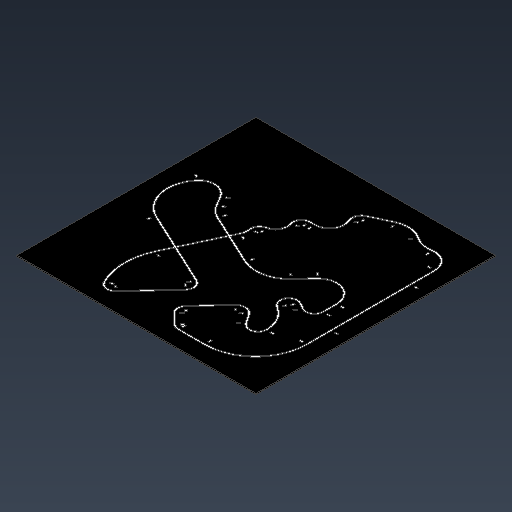
# Autodesk Inventor part: Pista_V2
Saved by Autodesk Inventor 2026.1 (Build 301233020, 233B)
## iProperties
Created: 2026-03-26
Part Number: Pista_V2
Material: Genérico
Document SubType Name: Modeling
Designer: celio
Density: 1 g/cm^3
Appearance: Padrão
Author: celio
Autodesk Inventor part; units mm, degrees
(part 1 of 2)
ref_plane "YZ Plane" through (0, 0, 0) normal (1, 0, 0) x (0, 1, 0)
ref_plane "XZ Plane" through (0, 0, 0) normal (0, 1, 0) x (-1, 0, 0)
ref_plane "XY Plane" through (0, 0, 0) normal (0, 0, 1) x (1, 0, 0)
sketch "Esboço3" plane through (0, 0, 0) normal (0, 1, 0) x (-1, 0, 0)
  line L0 (0, 0) -> (3000, 0)
  line L1 (3000, 0) -> (3000, 3000)
  line L2 (3000, 3000) -> (0, 3000)
  line L3 (0, 3000) -> (0, 0)
  line L4 (2800, 200) -> (200, 200)
  line L5 (200, 200) -> (200, 2800)
  line L6 (200, 2800) -> (2800, 2800)
  line L7 (2800, 2800) -> (2800, 200)
  dimension "d59" = 3000
  dimension "d60" = 3000
  dimension "d62" = 200
  constraints: 16 end point, 4 parallel, 2 perpendicular, 1 horizontal, 3 other
  measures "d59" distance of L2.end L1.end
  measures "d60" distance of L1.end L0.end
  measures "d62" distance between parallel lines of L0 L4
sketch "Esboço2" plane through (0, 0, 0) normal (0, 1, 0) x (-1, 0, 0)
  line L0 (203.1812, 1286.807) -> (200.7366, 822.1752)
  line L1 (200.7366, 822.1752) -> (213.5115, 423.3861)
  arc A0 (213.5115, 423.3861) -> (413.6397, 320.4728) centre (342.1557, 427.5072) ccw
  arc A1 (570.2436, 314.2066) -> (413.6397, 320.4728) centre (487.6339, 209.6798) ccw
  line L2 (570.2436, 314.2066) -> (674.3405, 236.4191)
  arc A2 (1219.6304, 696.5114) -> (1078.7214, 508.0068) centre (1224.6336, 545.8537) ccw
  line L3 (1219.6304, 696.5114) -> (1324.4415, 695.96)
  arc A3 (1324.4415, 695.96) -> (1397.9862, 805.8242) centre (1324.8585, 775.2288) ccw
  arc A4 (1495.576, 1001.8494) -> (1397.9862, 805.8242) centre (1531.4739, 861.6731) ccw
  arc A5 (1495.576, 1001.8494) -> (1575.056, 1115.5568) centre (1469.1771, 1104.9333) ccw
  arc A6 (1610.1393, 1248.5175) -> (1575.056, 1115.5568) centre (1770.3036, 1135.1473) ccw
  arc A7 (1610.1393, 1248.5175) -> (1897.3131, 1892.2335) centre (135.5939, 2292.255) ccw
  arc A8 (1897.3131, 1892.2335) -> (1829.6181, 2409.839) centre (1161.7229, 2059.2589) ccw
  arc A9 (1829.6181, 2409.839) -> (1693.1526, 2425.6392) centre (1755.9964, 2371.1948) ccw
  line L4 (1693.1526, 2425.6392) -> (1337.9343, 2057.7826)
  arc A10 (1337.9343, 2057.7826) -> (1380.2652, 1913.2849) centre (1400.2651, 1997.5932) ccw
  line L5 (1380.2652, 1913.2849) -> (1887.4115, 1728.4323)
  arc A11 (2119.9532, 1109.4728) -> (1887.4115, 1728.4323) centre (1738.2605, 1319.2342) ccw
  arc A12 (1975.2753, 1085.4597) -> (2119.9532, 1109.4728) centre (2038.1609, 1154.4223) ccw
  line L6 (1975.2753, 1085.4597) -> (1413.2086, 1508.9841)
  arc A13 (1413.2086, 1508.9841) -> (888.2123, 1444.7922) centre (1183.9822, 1204.7736) ccw
  line L7 (888.2123, 1444.7922) -> (778.9509, 1357.019)
  arc A14 (384.9481, 1573.1642) -> (778.9509, 1357.019) centre (626.66, 1546.5928) ccw
  line L8 (384.9481, 1573.1642) -> (401.2127, 1780.1036)
  arc A15 (504.1683, 1816.718) -> (401.2127, 1780.1036) centre (460.8686, 1775.4148) ccw
  line L9 (504.1683, 1816.718) -> (607.9366, 1732.0951)
  arc A16 (607.9366, 1732.0951) -> (741.3823, 1869.926) centre (668.7795, 1806.7034) ccw
  arc A17 (639.5829, 2333.3967) -> (741.3823, 1869.926) centre (1114.4343, 2194.7805) ccw
  arc A18 (732.3184, 2346.6255) -> (639.5829, 2333.3967) centre (688.9499, 2318.9857) ccw
  line L10 (732.3184, 2346.6255) -> (861.9261, 2116.7528)
  arc A19 (861.9261, 2116.7528) -> (1251.1364, 2088.539) centre (1065.8901, 2231.7525) ccw
  line L11 (1251.1364, 2088.539) -> (1508.7682, 2341.7211)
  arc A20 (1508.7682, 2341.7211) -> (1506.0798, 2440.9156) centre (1461.2572, 2390.0671) ccw
  line L12 (1506.0798, 2440.9156) -> (1393.2774, 2539.3529)
  arc A21 (1393.2774, 2539.3529) -> (1210.5735, 2615.666) centre (1187.4895, 2303.5341) ccw
  line L13 (1210.5735, 2615.666) -> (1002.8164, 2631.0309)
  arc A22 (1002.8164, 2631.0309) -> (552.19, 2393.7215) centre (967.3763, 2151.8265) ccw
  line L14 (552.19, 2393.7215) -> (332.983, 1988.7805)
  arc A23 (332.983, 1988.7805) -> (209.6535, 1597.6293) centre (1284.257, 1473.8266) ccw
  line L15 (209.6535, 1597.6293) -> (203.1812, 1286.807)
  arc A24 (674.3405, 236.4191) -> (867.7861, 220.3918) centre (783.8713, 382.9955) ccw
  line L16 (867.7861, 220.3918) -> (1017.5368, 282.8594)
  arc A25 (1017.5368, 282.8594) -> (1094.5203, 431.1081) centre (967.4227, 402.9955) ccw
  line L17 (1078.7214, 508.0068) -> (1094.5203, 431.1081)
  point P0 (0, 0)
  constraints: 52 point on circle, 36 end point, 26 centre point, 26 tangent
sketch "Esboço4" plane through (0, 0, 0) normal (0, 1, 0) x (-1, 0, 0)
  line L0 (213.5626, 543.4491) -> (213.5626, 2148.4491)
  line L1 (1237.817, 383.9797) -> (987.817, 267.4028)
  arc A0 (1237.817, 383.9797) -> (1294.7472, 540.3943) centre (1188.0748, 490.6521) ccw
  line L2 (1237.817, 383.9797) -> (1188.0748, 490.6521) construction
  line L3 (1294.7472, 540.3943) -> (1188.0748, 490.6521) construction
  arc A1 (1459.6046, 799.1685) -> (1294.7472, 540.3943) centre (1459.6046, 617.2685) ccw
  line L4 (1294.7472, 540.3943) -> (1459.6046, 617.2685) construction
  line L5 (1459.6046, 799.1685) -> (1459.6046, 617.2685) construction
  line L6 (1459.6046, 799.1685) -> (1523.8046, 799.1685)
  arc A2 (1523.8046, 799.1685) -> (1624.3517, 942.7647) centre (1523.8046, 906.1685) ccw
  line L7 (1523.8046, 799.1685) -> (1523.8046, 906.1685) construction
  line L8 (1624.3517, 942.7647) -> (1523.8046, 906.1685) construction
  arc A3 (1735.0069, 1134.425) -> (1624.3517, 942.7647) centre (1760.0903, 992.1695) ccw
  line L9 (1624.3517, 942.7647) -> (1760.0903, 992.1695) construction
  line L10 (1735.0069, 1134.425) -> (1760.0903, 992.1695) construction
  arc A4 (1735.0069, 1134.425) -> (1821.8009, 1258.3798) centre (1716.4265, 1239.7994) ccw
  line L11 (1735.0069, 1134.425) -> (1716.4265, 1239.7994) construction
  line L12 (1821.8009, 1258.3798) -> (1716.4265, 1239.7994) construction
  arc A5 (1835.2401, 1360.4606) -> (1821.8009, 1258.3798) centre (1990.4, 1288.1083) ccw
  line L13 (1821.8009, 1258.3798) -> (1990.4, 1288.1083) construction
  line L14 (1835.2401, 1360.4606) -> (1990.4, 1288.1083) construction
  line L15 (1835.2401, 1360.4606) -> (2094.6096, 1916.6801)
  arc A6 (2173.3347, 2085.5068) -> (2161.8741, 2742.0868) centre (1494.5102, 2402.0479) ccw
  line L16 (2173.3347, 2085.5068) -> (1494.5102, 2402.0479) construction
  line L17 (2161.8741, 2742.0868) -> (1494.5102, 2402.0479) construction
  arc A7 (2161.8741, 2742.0868) -> (1988.2816, 2766.4836) centre (2066.5364, 2693.5098) ccw
  line L18 (2161.8741, 2742.0868) -> (2066.5364, 2693.5098) construction
  line L19 (1988.2816, 2766.4836) -> (2066.5364, 2693.5098) construction
  line L20 (1988.2816, 2766.4836) -> (1568.6498, 2316.4836)
  arc A8 (1568.6498, 2316.4836) -> (1601.6845, 2146.5349) centre (1646.9046, 2243.5098) ccw
  line L21 (1568.6498, 2316.4836) -> (1646.9046, 2243.5098) construction
  line L22 (1601.6845, 2146.5349) -> (1646.9046, 2243.5098) construction
  line L23 (2541.6845, 1708.2057) -> (1601.6845, 2146.5349)
  arc A9 (2685.9234, 1057.5856) -> (2541.6845, 1708.2057) centre (2364.1848, 1327.5564) ccw
  line L24 (2541.6845, 1708.2057) -> (2364.1848, 1327.5564) construction
  line L25 (2685.9234, 1057.5856) -> (2364.1848, 1327.5564) construction
  arc A10 (2359.5095, 1086.1431) -> (2685.9234, 1057.5856) centre (2532.7146, 1186.1431) ccw
  line L26 (2685.9234, 1057.5856) -> (2532.7146, 1186.1431) construction
  line L27 (2359.5095, 1086.1431) -> (2532.7146, 1186.1431) construction
  arc A11 (1507.2053, 1631.1354) -> (1022.5371, 1536.9255) centre (1329.7056, 1250.4862) ccw
  line L28 (1507.2053, 1631.1354) -> (1329.7056, 1250.4862) construction
  line L29 (1022.5371, 1536.9255) -> (1329.7056, 1250.4862) construction
  line L30 (1022.5371, 1536.9255) -> (862.6577, 1365.4758)
  arc A12 (464.4463, 1522.3354) -> (862.6577, 1365.4758) centre (694.4463, 1522.3354) ccw
  line L31 (862.6577, 1365.4758) -> (694.4463, 1522.3354) construction
  line L32 (464.4463, 1522.3354) -> (694.4463, 1522.3354) construction
  line L33 (464.4463, 1522.3354) -> (464.4463, 1693.5354)
  arc A13 (624.9463, 1786.2002) -> (464.4463, 1693.5354) centre (571.4463, 1693.5354) ccw
  line L34 (464.4463, 1693.5354) -> (571.4463, 1693.5354) construction
  line L35 (624.9463, 1786.2002) -> (571.4463, 1693.5354) construction
  line L36 (624.9463, 1786.2002) -> (699.8463, 1742.9566)
  arc A14 (699.8463, 1742.9566) -> (806.8463, 1928.2861) centre (753.3463, 1835.6213) ccw
  line L37 (699.8463, 1742.9566) -> (753.3463, 1835.6213) construction
  line L38 (806.8463, 1928.2861) -> (753.3463, 1835.6213) construction
  arc A15 (624.9463, 2243.3461) -> (806.8463, 1928.2861) centre (988.7463, 2243.3461) ccw
  line L39 (806.8463, 1928.2861) -> (988.7463, 2243.3461) construction
  line L40 (624.9463, 2243.3461) -> (988.7463, 2243.3461) construction
  arc A16 (819.5956, 2304.7188) -> (624.9463, 2243.3461) centre (731.9463, 2243.3461) ccw
  line L41 (624.9463, 2243.3461) -> (731.9463, 2243.3461) construction
  line L42 (819.5956, 2304.7188) -> (731.9463, 2243.3461) construction
  line L43 (819.5956, 2304.7188) -> (905.1956, 2182.4693)
  arc A17 (905.1956, 2182.4693) -> (1091.2563, 2169.4587) centre (1003.4939, 2251.2985) ccw
  line L44 (905.1956, 2182.4693) -> (1003.4939, 2251.2985) construction
  line L45 (1091.2563, 2169.4587) -> (1003.4939, 2251.2985) construction
  line L46 (1091.2563, 2169.4587) -> (1390.8563, 2490.7403)
  arc A18 (1390.8563, 2490.7403) -> (1385.5753, 2641.969) centre (1312.6015, 2563.7142) ccw
  line L47 (1390.8563, 2490.7403) -> (1312.6015, 2563.7142) construction
  line L48 (1385.5753, 2641.969) -> (1312.6015, 2563.7142) construction
  line L49 (1385.5753, 2641.969) -> (1257.1753, 2761.704)
  arc A19 (1257.1753, 2761.704) -> (1184.2015, 2790.4491) centre (1184.2015, 2683.4491) ccw
  line L50 (1257.1753, 2761.704) -> (1184.2015, 2683.4491) construction
  line L51 (1184.2015, 2790.4491) -> (1184.2015, 2683.4491) construction
  line L52 (1184.2015, 2790.4491) -> (855.5626, 2790.4491)
  arc A20 (855.5626, 2790.4491) -> (213.5626, 2148.4491) centre (855.5626, 2148.4491) ccw
  line L53 (213.5626, 2148.4491) -> (855.5626, 2148.4491) construction
  line L54 (855.5626, 2790.4491) -> (855.5626, 2148.4491) construction
  arc A21 (213.5626, 543.4491) -> (452.1653, 343.2377) centre (416.8626, 543.4491) ccw
  line L55 (213.5626, 543.4491) -> (416.8626, 543.4491) construction
  line L56 (452.1653, 343.2377) -> (416.8626, 543.4491) construction
  arc A22 (668.0385, 295.3798) -> (452.1653, 343.2377) centre (502.3323, 58.7267) ccw
  line L57 (452.1653, 343.2377) -> (502.3323, 58.7267) construction
  line L58 (668.0385, 295.3798) -> (502.3323, 58.7267) construction
  arc A23 (668.0385, 295.3798) -> (987.817, 267.4028) centre (852.1565, 558.3276) ccw
  line L59 (1507.2053, 1631.1354) -> (1880.3256, 1457.1466)
  line L60 (2359.5095, 1086.1431) -> (2290.2274, 1206.1431)
  arc A24 (2290.2274, 1206.1431) -> (2157.2053, 1328.0354) centre (2030.4198, 1056.1431) ccw
  line L61 (2290.2274, 1206.1431) -> (2030.4198, 1056.1431) construction
  line L62 (2030.4198, 1056.1431) -> (2157.2053, 1328.0354) construction
  line L63 (987.817, 267.4028) -> (852.1565, 558.3276) construction
  line L64 (852.1565, 558.3276) -> (668.0385, 295.3798) construction
  line L65 (2094.6096, 1916.6801) -> (2173.3347, 2085.5068)
  line L66 (1880.3256, 1457.1466) -> (2157.2053, 1328.0354)
  point P0 (0, 0)
  dimension "d63" = 1605
  dimension "d74" = 117.7
  dimension "d75" = 90
  dimension "d76" = 181.9
  dimension "d77" = 115
  dimension "d78" = 64.2
  dimension "d79" = 107
  dimension "d80" = 110
  dimension "d81" = 144.45
  dimension "d82" = 100
  dimension "d83" = 107
  dimension "d84" = 90
  dimension "d85" = 171.2
  dimension "d86" = 35
  dimension "d87" = 800
  dimension "d88" = 749
  dimension "d90" = 107
  dimension "d91" = 110
  dimension "d92" = 450
  dimension "d93" = 107
  dimension "d94" = 108
  dimension "d96" = 420
  dimension "d97" = 105
  dimension "d98" = 200
  dimension "d99" = 110
  dimension "d101" = 420
  dimension "d102" = 72
  dimension "d103" = 230
  dimension "d104" = 137
  dimension "d106" = 171.2
  dimension "d107" = 107
  dimension "d109" = 74.9
  dimension "d110" = 107
  dimension "d111" = 180
  dimension "d112" = 363.8
  dimension "d113" = 60
  dimension "d114" = 107
  dimension "d115" = 145
  dimension "d116" = 85.6
  dimension "d117" = 120
  dimension "d119" = 299.6
  dimension "d120" = 107
  dimension "d121" = 90
  dimension "d122" = 128.4
  dimension "d123" = 107
  dimension "d124" = 43
  dimension "d126" = 642
  dimension "d127" = 90
  dimension "d129" = 328.6388
  dimension "d131" = 203.3
  dimension "d132" = 100
  dimension "d133" = 288.9
  dimension "d134" = 45
  dimension "d137" = 250
  dimension "d138" = 321
  dimension "d141" = 300
  dimension "d143" = 940
  dimension "d144" = 120
  dimension "d146" = 120
  dimension "d147" = 650
  dimension "d148" = 248.8727
  dimension "d149" = 250.8837
  dimension "d150" = 60
  constraints: 134 end point, 50 point on circle, 28 tangent, 25 centre point, 21 perpendicular, 2 point on line, 2 vertical, 1 collinear, 1 parallel
  measures "d63" distance of L0.start L0.end
  measures "d74" radius of A0
  measures "d75" angle of L2 L3
  measures "d76" radius of A1
  measures "d77" angle of L5 L4
  measures "d78" distance of L5.start L6.end
  measures "d79" radius of A2
  measures "d80" angle of L7 L8
  measures "d81" radius of A3
  measures "d82" angle of L10 L9
  measures "d83" radius of A4
  measures "d84" angle of L11 L12
  measures "d85" radius of A5
  measures "d86" angle of L14 L13
  measures "d87" distance of L14.start L16.start
  measures "d88" radius of A6
  measures "d90" radius of A7
  measures "d91" angle of L18 L19
  measures "d92" vertical distance of L19.start L20.end
  measures "d93" radius of A8
  measures "d94" angle of L21 L22
  measures "d96" radius of A9
  measures "d97" angle of L25 L24
  measures "d98" radius of A10
  measures "d99" angle of L27 L26
  measures "d101" radius of A11
  measures "d102" angle of L28 L29
  measures "d103" radius of A12
  measures "d104" angle of L32 L31
  measures "d106" distance of L32.start L33.end
  measures "d107" radius of A13
  measures "d109" horizontal distance of L35.start L36.end
  measures "d110" radius of A14
  measures "d111" angle of L37 L38
  measures "d112" radius of A15
  measures "d113" angle of L40 L39
  measures "d114" radius of A16
  measures "d115" angle of L42 L41
  measures "d116" horizontal distance of L42.start L43.end
  measures "d117" radius of A17
  measures "d119" horizontal distance of L45.start L46.end
  measures "d120" radius of A18
  measures "d121" angle of L47 L48
  measures "d122" horizontal distance of L48.start L49.end
  measures "d123" radius of A19
  measures "d124" angle of L50 L51
  measures "d126" radius of A20
  measures "d127" angle of L54 L53
  measures "d129" distance of L51.start L52.end
  measures "d131" radius of A21
  measures "d132" angle of L55 L56
  measures "d133" radius of A22
  measures "d134" angle of L58 L57
  measures "d137" horizontal distance of L1.start L1.end
  measures "d138" radius of A23
  measures "d141" radius of A24
  measures "d143" horizontal distance of L23.start L22.start
  measures "d144" angle of L34 L35
  measures "d146" vertical distance of L27.start L60.end
  measures "d147" horizontal distance of L28.start L62.end
  measures "d148" distance between parallel lines of L20 L46
  measures "d149" distance from line of L0 L32.start
  measures "d150" angle of L63 L64
sketch "Esboço5" plane through (0, 0, 0) normal (0, 1, 0) x (-1, 0, 0)
  arc A0 (699.8463, 1742.9566) -> (806.8463, 1928.2861) centre (753.3463, 1835.6213) ccw projected
  line L0 (1022.5371, 1536.9255) -> (862.6577, 1365.4758) projected
  arc A1 (1459.6046, 799.1685) -> (1294.7472, 540.3943) centre (1459.6046, 617.2685) ccw projected
  arc A2 (1237.817, 383.9797) -> (1294.7472, 540.3943) centre (1188.0748, 490.6521) ccw projected
  line L1 (624.9463, 1786.2002) -> (699.8463, 1742.9566) projected
  arc A3 (624.9463, 1786.2002) -> (464.4463, 1693.5354) centre (571.4463, 1693.5354) ccw projected
  arc A4 (464.4463, 1522.3354) -> (862.6577, 1365.4758) centre (694.4463, 1522.3354) ccw projected
  line L2 (464.4463, 1522.3354) -> (464.4463, 1693.5354) projected
  line L3 (213.5626, 543.4491) -> (213.5626, 2148.4491) projected
  arc A5 (624.9463, 2243.3461) -> (806.8463, 1928.2861) centre (988.7463, 2243.3461) ccw projected
  line L4 (819.5956, 2304.7188) -> (905.1956, 2182.4693) projected
  arc A6 (819.5956, 2304.7188) -> (624.9463, 2243.3461) centre (731.9463, 2243.3461) ccw projected
  arc A7 (855.5626, 2790.4491) -> (213.5626, 2148.4491) centre (855.5626, 2148.4491) ccw projected
  arc A8 (1390.8563, 2490.7403) -> (1385.5753, 2641.969) centre (1312.6015, 2563.7142) ccw projected
  line L5 (1385.5753, 2641.969) -> (1257.1753, 2761.704) projected
  arc A9 (1257.1753, 2761.704) -> (1184.2015, 2790.4491) centre (1184.2015, 2683.4491) ccw projected
  line L6 (1091.2563, 2169.4587) -> (1390.8563, 2490.7403) projected
  arc A10 (905.1956, 2182.4693) -> (1091.2563, 2169.4587) centre (1003.4939, 2251.2985) ccw projected
  line L7 (1184.2015, 2790.4491) -> (855.5626, 2790.4491) projected
  line L8 (1237.817, 383.9797) -> (987.817, 267.4028) projected
  arc A11 (668.0385, 295.3798) -> (987.817, 267.4028) centre (852.1565, 558.3276) ccw projected
  arc A12 (668.0385, 295.3798) -> (452.1653, 343.2377) centre (502.3323, 58.7267) ccw projected
  arc A13 (213.5626, 543.4491) -> (452.1653, 343.2377) centre (416.8626, 543.4491) ccw projected
  arc A14 (1507.2053, 1631.1354) -> (1022.5371, 1536.9255) centre (1329.7056, 1250.4862) ccw projected
  line L9 (1507.2053, 1631.1354) -> (1880.3256, 1457.1466) projected
  arc A15 (1835.2401, 1360.4606) -> (1821.8009, 1258.3798) centre (1990.4, 1288.1083) ccw projected
  arc A16 (1735.0069, 1134.425) -> (1821.8009, 1258.3798) centre (1716.4265, 1239.7994) ccw projected
  line L10 (1459.6046, 799.1685) -> (1523.8046, 799.1685) projected
  arc A17 (1523.8046, 799.1685) -> (1624.3517, 942.7647) centre (1523.8046, 906.1685) ccw projected
  arc A18 (1735.0069, 1134.425) -> (1624.3517, 942.7647) centre (1760.0903, 992.1695) ccw projected
  line L11 (1880.3256, 1457.1466) -> (1835.2401, 1360.4606)
  arc A19 (1523.8046, 809.1685) -> (1614.9548, 939.3445) centre (1523.8046, 906.1685) ccw
  line L12 (1523.8046, 809.1685) -> (1459.6046, 809.1685)
  arc A20 (1459.6046, 809.1685) -> (1285.6842, 536.1681) centre (1459.6046, 617.2685) ccw
  arc A21 (1233.5908, 393.0428) -> (1285.6842, 536.1681) centre (1188.0748, 490.6521) ccw
  line L13 (1233.5908, 393.0428) -> (983.5908, 276.4658)
  arc A22 (673.7743, 303.5713) -> (983.5908, 276.4658) centre (852.1565, 558.3276) ccw
  arc A23 (673.7743, 303.5713) -> (450.4288, 353.0858) centre (502.3323, 58.7267) ccw
  arc A24 (223.5626, 543.4491) -> (450.4288, 353.0858) centre (416.8626, 543.4491) ccw
  line L14 (223.5626, 543.4491) -> (223.5626, 2148.4491)
  arc A25 (855.5626, 2780.4491) -> (223.5626, 2148.4491) centre (855.5626, 2148.4491) ccw
  line L15 (855.5626, 2780.4491) -> (1184.2015, 2780.4491)
  arc A26 (1250.3553, 2754.3904) -> (1184.2015, 2780.4491) centre (1184.2015, 2683.4491) ccw
  line L16 (1250.3553, 2754.3904) -> (1378.7553, 2634.6555)
  arc A27 (1383.5428, 2497.5603) -> (1378.7553, 2634.6555) centre (1312.6015, 2563.7142) ccw
  line L17 (1383.5428, 2497.5603) -> (1083.9428, 2176.2787)
  arc A28 (913.3871, 2188.2051) -> (1083.9428, 2176.2787) centre (1003.4939, 2251.2985) ccw
  line L18 (913.3871, 2188.2051) -> (827.7871, 2310.4545)
  arc A29 (827.7871, 2310.4545) -> (614.9463, 2243.3461) centre (731.9463, 2243.3461) ccw
  arc A30 (614.9463, 2243.3461) -> (801.8463, 1919.6258) centre (988.7463, 2243.3461) ccw
  arc A31 (704.8463, 1751.6169) -> (801.8463, 1919.6258) centre (753.3463, 1835.6213) ccw
  line L19 (704.8463, 1751.6169) -> (629.9463, 1794.8604)
  arc A32 (629.9463, 1794.8604) -> (454.4463, 1693.5354) centre (571.4463, 1693.5354) ccw
  line L20 (454.4463, 1693.5354) -> (454.4463, 1522.3354)
  arc A33 (454.4463, 1522.3354) -> (869.9712, 1358.6558) centre (694.4463, 1522.3354) ccw
  line L21 (869.9712, 1358.6558) -> (1029.8506, 1530.1055)
  arc A34 (1502.9791, 1622.0723) -> (1029.8506, 1530.1055) centre (1329.7056, 1250.4862) ccw
  line L22 (1502.9791, 1622.0723) -> (1867.0363, 1452.3097)
  line L23 (1867.0363, 1452.3097) -> (1826.1771, 1364.6868)
  arc A35 (1826.1771, 1364.6868) -> (1811.9529, 1256.6433) centre (1990.4, 1288.1083) ccw
  arc A36 (1733.2704, 1144.2731) -> (1811.9529, 1256.6433) centre (1716.4265, 1239.7994) ccw
  arc A37 (1733.2704, 1144.2731) -> (1614.9548, 939.3445) centre (1760.0903, 992.1695) ccw
  arc A38 (1523.8046, 789.1685) -> (1633.7487, 946.1849) centre (1523.8046, 906.1685) ccw
  line L24 (1523.8046, 789.1685) -> (1459.6046, 789.1685)
  arc A39 (1459.6046, 789.1685) -> (1303.8103, 544.6205) centre (1459.6046, 617.2685) ccw
  arc A40 (1242.0432, 374.9166) -> (1303.8103, 544.6205) centre (1188.0748, 490.6521) ccw
  line L25 (1242.0432, 374.9166) -> (992.0432, 258.3397)
  arc A41 (662.3027, 287.1882) -> (992.0432, 258.3397) centre (852.1565, 558.3276) ccw
  arc A42 (662.3027, 287.1882) -> (453.9018, 333.3896) centre (502.3323, 58.7267) ccw
  arc A43 (203.5626, 543.4491) -> (453.9018, 333.3896) centre (416.8626, 543.4491) ccw
  line L26 (203.5626, 543.4491) -> (203.5626, 2148.4491)
  arc A44 (855.5626, 2800.4491) -> (203.5626, 2148.4491) centre (855.5626, 2148.4491) ccw
  line L27 (855.5626, 2800.4491) -> (1184.2015, 2800.4491)
  arc A45 (1263.9953, 2769.0175) -> (1184.2015, 2800.4491) centre (1184.2015, 2683.4491) ccw
  line L28 (1263.9953, 2769.0175) -> (1392.3953, 2649.2826)
  arc A46 (1398.1698, 2483.9204) -> (1392.3953, 2649.2826) centre (1312.6015, 2563.7142) ccw
  line L29 (1398.1698, 2483.9204) -> (1098.5698, 2162.6387)
  arc A47 (897.0041, 2176.7335) -> (1098.5698, 2162.6387) centre (1003.4939, 2251.2985) ccw
  line L30 (897.0041, 2176.7335) -> (811.4041, 2298.983)
  arc A48 (811.4041, 2298.983) -> (634.9463, 2243.3461) centre (731.9463, 2243.3461) ccw
  arc A49 (634.9463, 2243.3461) -> (811.8463, 1936.9463) centre (988.7463, 2243.3461) ccw
  arc A50 (694.8463, 1734.2964) -> (811.8463, 1936.9463) centre (753.3463, 1835.6213) ccw
  line L31 (694.8463, 1734.2964) -> (619.9463, 1777.5399)
  arc A51 (619.9463, 1777.5399) -> (474.4463, 1693.5354) centre (571.4463, 1693.5354) ccw
  line L32 (474.4463, 1693.5354) -> (474.4463, 1522.3354)
  arc A52 (474.4463, 1522.3354) -> (855.3442, 1372.2958) centre (694.4463, 1522.3354) ccw
  line L33 (855.3442, 1372.2958) -> (1015.2235, 1543.7454)
  arc A53 (1511.4315, 1640.1985) -> (1015.2235, 1543.7454) centre (1329.7056, 1250.4862) ccw
  line L34 (1511.4315, 1640.1985) -> (1893.6148, 1461.9835)
  line L35 (1893.6148, 1461.9835) -> (1844.3032, 1356.2344)
  arc A54 (1844.3032, 1356.2344) -> (1831.649, 1260.1162) centre (1990.4, 1288.1083) ccw
  arc A55 (1736.7433, 1124.5769) -> (1831.649, 1260.1162) centre (1716.4265, 1239.7994) ccw
  arc A56 (1736.7433, 1124.5769) -> (1633.7487, 946.1849) centre (1760.0903, 992.1695) ccw
  line L36 (2094.6096, 1916.6801) -> (2173.3347, 2085.5068) projected
  arc A57 (2173.3347, 2085.5068) -> (2161.8741, 2742.0868) centre (1494.5102, 2402.0479) ccw projected
  arc A58 (2161.8741, 2742.0868) -> (1988.2816, 2766.4836) centre (2066.5364, 2693.5098) ccw projected
  line L37 (1988.2816, 2766.4836) -> (1568.6498, 2316.4836) projected
  arc A59 (1568.6498, 2316.4836) -> (1601.6845, 2146.5349) centre (1646.9046, 2243.5098) ccw projected
  line L38 (2094.6096, 1916.6801) -> (1601.6845, 2146.5349)
  arc A60 (1575.9633, 2309.6636) -> (1605.9106, 2155.5979) centre (1646.9046, 2243.5098) ccw
  line L39 (1575.9633, 2309.6636) -> (1995.5951, 2759.6636)
  arc A61 (2152.964, 2737.5469) -> (1995.5951, 2759.6636) centre (2066.5364, 2693.5098) ccw
  arc A62 (2164.2717, 2089.733) -> (2152.964, 2737.5469) centre (1494.5102, 2402.0479) ccw
  line L40 (2164.2717, 2089.733) -> (2089.7727, 1929.9694)
  line L41 (2089.7727, 1929.9694) -> (1605.9106, 2155.5979)
  arc A63 (1561.3362, 2323.3036) -> (1597.4583, 2137.4718) centre (1646.9046, 2243.5098) ccw
  line L42 (1561.3362, 2323.3036) -> (1980.968, 2773.3036)
  arc A64 (2170.7842, 2746.6267) -> (1980.968, 2773.3036) centre (2066.5364, 2693.5098) ccw
  arc A65 (2182.3978, 2081.2806) -> (2170.7842, 2746.6267) centre (1494.5102, 2402.0479) ccw
  line L43 (2182.3978, 2081.2806) -> (2099.4465, 1903.3908)
  line L44 (2099.4465, 1903.3908) -> (1597.4583, 2137.4718)
  arc A66 (2685.9234, 1057.5856) -> (2541.6845, 1708.2057) centre (2364.1848, 1327.5564) ccw projected
  arc A67 (2359.5095, 1086.1431) -> (2685.9234, 1057.5856) centre (2532.7146, 1186.1431) ccw projected
  line L45 (2359.5095, 1086.1431) -> (2290.2274, 1206.1431) projected
  arc A68 (2290.2274, 1206.1431) -> (2157.2053, 1328.0354) centre (2030.4198, 1056.1431) ccw projected
  line L46 (2541.6845, 1708.2057) -> (2094.6096, 1916.6801)
  line L47 (2157.2053, 1328.0354) -> (1880.3256, 1457.1466)
  line L48 (1844.3032, 1356.2344) -> (1885.1625, 1443.8573)
  line L49 (1885.1625, 1443.8573) -> (2152.9791, 1318.9724)
  arc A69 (2281.5672, 1201.1431) -> (2152.9791, 1318.9724) centre (2030.4198, 1056.1431) ccw
  line L50 (2281.5672, 1201.1431) -> (2350.8492, 1081.1431)
  arc A70 (2350.8492, 1081.1431) -> (2693.5839, 1051.1577) centre (2532.7146, 1186.1431) ccw
  arc A71 (2693.5839, 1051.1577) -> (2545.9106, 1717.2687) centre (2364.1848, 1327.5564) ccw
  line L51 (2545.9106, 1717.2687) -> (2098.8357, 1925.7432)
  line L52 (1826.1771, 1364.6868) -> (1875.4887, 1470.4359)
  line L53 (1875.4887, 1470.4359) -> (2161.4315, 1337.0985)
  arc A72 (2298.8877, 1211.1431) -> (2161.4315, 1337.0985) centre (2030.4198, 1056.1431) ccw
  line L54 (2298.8877, 1211.1431) -> (2368.1697, 1091.1431)
  arc A73 (2368.1697, 1091.1431) -> (2678.263, 1064.0135) centre (2532.7146, 1186.1431) ccw
  arc A74 (2678.263, 1064.0135) -> (2537.4583, 1699.1426) centre (2364.1848, 1327.5564) ccw
  line L55 (2537.4583, 1699.1426) -> (2090.3834, 1907.617)
  line L56 (2094.6096, 1916.6801) -> (1880.3256, 1457.1466)
  line L57 (2103.6726, 1912.4539) -> (1889.3886, 1452.9204)
  line L58 (2085.5465, 1920.9063) -> (1871.2625, 1461.3728)
  point P0 (2107.8988, 1921.517)
  point P1 (2081.3203, 1911.8432)
  dimension "d151" = 10
  dimension "d152" = 10
  dimension "d153" = 10
  dimension "d154" = 10
  dimension "d155" = 10
  dimension "d156" = 10
  dimension "d157" = 10
  dimension "d158" = 10
  constraints: 100 point on circle, 90 end point, 50 centre point, 4 perpendicular, 2 parallel, 1 collinear, 1 tangent, 82 other
  measures "d151" radial gap between concentric circles of A17 A19
  measures "d152" radial gap between concentric circles of A17 A38
  measures "d153" distance between parallel lines of L38 L41
  measures "d154" distance between parallel lines of L38 L44
  measures "d155" distance between parallel lines of L47 L49
  measures "d156" distance between parallel lines of L47 L53
  measures "d157" distance between parallel lines of L56 L57
  measures "d158" distance between parallel lines of L56 L58
sketch "Esboço6" plane through (0, 0, 0) normal (0, 1, 0) x (-1, 0, 0)
  line L0 (213.5626, 2148.4491) -> (855.5626, 2148.4491) construction
  line L1 (855.5626, 2790.4491) -> (855.5626, 2148.4491) construction
  line L2 (1184.2015, 2790.4491) -> (1184.2015, 2683.4491) construction
  line L3 (1257.1753, 2761.704) -> (1184.2015, 2683.4491) construction
  line L4 (1385.5753, 2641.969) -> (1312.6015, 2563.7142) construction
  line L5 (1390.8563, 2490.7403) -> (1312.6015, 2563.7142) construction
  line L6 (905.1956, 2182.4693) -> (1003.4939, 2251.2985) construction
  line L7 (1091.2563, 2169.4587) -> (1003.4939, 2251.2985) construction
  line L8 (819.5956, 2304.7188) -> (731.9463, 2243.3461) construction
  line L9 (624.9463, 2243.3461) -> (988.7463, 2243.3461) construction
  line L10 (806.8463, 1928.2861) -> (988.7463, 2243.3461) construction
  line L11 (806.8463, 1928.2861) -> (753.3463, 1835.6213) construction
  line L12 (699.8463, 1742.9566) -> (753.3463, 1835.6213) construction
  line L13 (624.9463, 1786.2002) -> (571.4463, 1693.5354) construction
  line L14 (464.4463, 1693.5354) -> (571.4463, 1693.5354) construction
  line L15 (464.4463, 1522.3354) -> (694.4463, 1522.3354) construction
  line L16 (862.6577, 1365.4758) -> (694.4463, 1522.3354) construction
  line L17 (1507.2053, 1631.1354) -> (1329.7056, 1250.4862) construction
  line L18 (1022.5371, 1536.9255) -> (1329.7056, 1250.4862) construction
  line L19 (1601.6845, 2146.5349) -> (1646.9046, 2243.5098) construction
  line L20 (1568.6498, 2316.4836) -> (1646.9046, 2243.5098) construction
  line L21 (2173.3347, 2085.5068) -> (1494.5102, 2402.0479) construction
  line L22 (2161.8741, 2742.0868) -> (1494.5102, 2402.0479) construction
  line L23 (1988.2816, 2766.4836) -> (2066.5364, 2693.5098) construction
  line L24 (1835.2401, 1360.4606) -> (1990.4, 1288.1083) construction
  line L25 (1821.8009, 1258.3798) -> (1990.4, 1288.1083) construction
  line L26 (1735.0069, 1134.425) -> (1716.4265, 1239.7994) construction
  line L27 (1821.8009, 1258.3798) -> (1716.4265, 1239.7994) construction
  line L28 (1735.0069, 1134.425) -> (1760.0903, 992.1695) construction
  line L29 (1624.3517, 942.7647) -> (1760.0903, 992.1695) construction
  line L30 (1624.3517, 942.7647) -> (1523.8046, 906.1685) construction
  line L31 (1523.8046, 799.1685) -> (1523.8046, 906.1685) construction
  line L32 (1459.6046, 799.1685) -> (1459.6046, 617.2685) construction
  line L33 (1294.7472, 540.3943) -> (1459.6046, 617.2685) construction
  line L34 (1294.7472, 540.3943) -> (1188.0748, 490.6521) construction
  line L35 (1237.817, 383.9797) -> (1188.0748, 490.6521) construction
  line L36 (987.817, 267.4028) -> (852.1565, 558.3276) construction
  line L37 (852.1565, 558.3276) -> (668.0385, 295.3798) construction
  line L38 (452.1653, 343.2377) -> (502.3323, 58.7267) construction
  line L39 (668.0385, 295.3798) -> (502.3323, 58.7267) construction
  line L40 (452.1653, 343.2377) -> (416.8626, 543.4491) construction
  line L41 (213.5626, 543.4491) -> (416.8626, 543.4491) construction
  line L42 (2541.6845, 1708.2057) -> (2364.1848, 1327.5564) construction
  line L43 (2685.9234, 1057.5856) -> (2364.1848, 1327.5564) construction
  line L44 (2359.5095, 1086.1431) -> (2532.7146, 1186.1431) construction
  line L45 (2290.2274, 1206.1431) -> (2030.4198, 1056.1431) construction
  line L46 (2030.4198, 1056.1431) -> (2157.2053, 1328.0354) construction
  line L47 (263.5626, 533.4491) -> (303.5626, 533.4491)
  line L48 (303.5626, 533.4491) -> (303.5626, 553.4491)
  line L49 (303.5626, 553.4491) -> (263.5626, 553.4491)
  line L50 (263.5626, 553.4491) -> (263.5626, 533.4491)
  line L51 (263.5626, 533.4491) -> (303.5626, 553.4491) construction
  line L52 (303.5626, 533.4491) -> (263.5626, 553.4491) construction
  line L53 (426.6889, 430.1339) -> (446.385, 433.6069)
  line L54 (446.385, 433.6069) -> (453.331, 394.2146)
  line L55 (453.331, 394.2146) -> (433.6348, 390.7416)
  line L56 (433.6348, 390.7416) -> (426.6889, 430.1339)
  line L57 (426.6889, 430.1339) -> (453.331, 394.2146) construction
  line L58 (446.385, 433.6069) -> (433.6348, 390.7416) construction
  line L59 (704.9088, 330.6016) -> (688.5258, 342.0731)
  line L60 (688.5258, 342.0731) -> (711.4688, 374.8392)
  line L61 (711.4688, 374.8392) -> (727.8519, 363.3677)
  line L62 (727.8519, 363.3677) -> (704.9088, 330.6016)
  line L63 (704.9088, 330.6016) -> (711.4688, 374.8392) construction
  line L64 (688.5258, 342.0731) -> (727.8519, 363.3677) construction
  line L65 (957.623, 308.492) -> (975.7492, 316.9443)
  line L66 (975.7492, 316.9443) -> (958.8444, 353.1966)
  line L67 (958.8444, 353.1966) -> (940.7183, 344.7443)
  line L68 (940.7183, 344.7443) -> (957.623, 308.492)
  line L69 (957.623, 308.492) -> (958.8444, 353.1966) construction
  line L70 (975.7492, 316.9443) -> (940.7183, 344.7443) construction
  line L71 (1208.8444, 469.7736) -> (1190.7183, 461.3212)
  line L72 (1190.7183, 461.3212) -> (1207.623, 425.0689)
  line L73 (1207.623, 425.0689) -> (1225.7492, 433.5212)
  line L74 (1225.7492, 433.5212) -> (1208.8444, 469.7736)
  line L75 (1208.8444, 469.7736) -> (1207.623, 425.0689) construction
  line L76 (1190.7183, 461.3212) -> (1225.7492, 433.5212) construction
  line L77 (1208.9534, 511.4217) -> (1245.2057, 528.3264)
  line L78 (1245.2057, 528.3264) -> (1253.658, 510.2003)
  line L79 (1253.658, 510.2003) -> (1217.4057, 493.2956)
  line L80 (1217.4057, 493.2956) -> (1208.9534, 511.4217)
  line L81 (1208.9534, 511.4217) -> (1253.658, 510.2003) construction
  line L82 (1245.2057, 528.3264) -> (1217.4057, 493.2956) construction
  line L83 (1459.6046, 617.2685) -> (1459.6046, 898.9769) construction
  line L84 (1449.6046, 849.1685) -> (1469.6046, 849.1685)
  line L85 (1469.6046, 849.1685) -> (1469.6046, 889.1685)
  line L86 (1469.6046, 889.1685) -> (1449.6046, 889.1685)
  line L87 (1449.6046, 889.1685) -> (1449.6046, 849.1685)
  line L88 (1449.6046, 849.1685) -> (1469.6046, 889.1685) construction
  line L89 (1469.6046, 849.1685) -> (1449.6046, 889.1685) construction
  line L90 (1513.8046, 889.1685) -> (1533.8046, 889.1685)
  line L91 (1533.8046, 889.1685) -> (1533.8046, 849.1685)
  line L92 (1533.8046, 849.1685) -> (1513.8046, 849.1685)
  line L93 (1513.8046, 849.1685) -> (1513.8046, 889.1685)
  line L94 (1513.8046, 889.1685) -> (1533.8046, 849.1685) construction
  line L95 (1533.8046, 889.1685) -> (1513.8046, 849.1685) construction
  line L96 (1580.7873, 916.2668) -> (1543.1996, 902.586)
  line L97 (1543.1996, 902.586) -> (1536.3592, 921.3798)
  line L98 (1536.3592, 921.3798) -> (1573.9469, 935.0606)
  line L99 (1573.9469, 935.0606) -> (1580.7873, 916.2668)
  line L100 (1580.7873, 916.2668) -> (1536.3592, 921.3798) construction
  line L101 (1543.1996, 902.586) -> (1573.9469, 935.0606) construction
  line L102 (1709.5304, 1221.3212) -> (1729.2266, 1224.7942)
  line L103 (1729.2266, 1224.7942) -> (1736.1725, 1185.4019)
  line L104 (1736.1725, 1185.4019) -> (1716.4764, 1181.9289)
  line L105 (1716.4764, 1181.9289) -> (1709.5304, 1221.3212)
  line L106 (1709.5304, 1221.3212) -> (1736.1725, 1185.4019) construction
  line L107 (1729.2266, 1224.7942) -> (1716.4764, 1181.9289) construction
  line L108 (1774.297, 1239.8493) -> (1734.9047, 1232.9034)
  line L109 (1734.9047, 1232.9034) -> (1731.4318, 1252.5995)
  line L110 (1731.4318, 1252.5995) -> (1770.8241, 1259.5454)
  line L111 (1770.8241, 1259.5454) -> (1774.297, 1239.8493)
  line L112 (1774.297, 1239.8493) -> (1731.4318, 1252.5995) construction
  line L113 (1734.9047, 1232.9034) -> (1770.8241, 1259.5454) construction
  line L114 (1990.4, 1288.1083) -> (1734.37, 1408.6992) construction
  line L115 (1749.8392, 1390.3594) -> (1786.0262, 1373.3153)
  line L116 (1786.0262, 1373.3153) -> (1794.5483, 1391.4088)
  line L117 (1794.5483, 1391.4088) -> (1758.3613, 1408.4529)
  line L118 (1758.3613, 1408.4529) -> (1749.8392, 1390.3594)
  line L119 (1749.8392, 1390.3594) -> (1794.5483, 1391.4088) construction
  line L120 (1786.0262, 1373.3153) -> (1758.3613, 1408.4529) construction
  line L121 (2087.5409, 2114.4794) -> (2123.7932, 2097.5746)
  line L122 (2123.7932, 2097.5746) -> (2132.2455, 2115.7008)
  line L123 (2132.2455, 2115.7008) -> (2095.9932, 2132.6055)
  line L124 (2095.9932, 2132.6055) -> (2087.5409, 2114.4794)
  line L125 (2087.5409, 2114.4794) -> (2132.2455, 2115.7008) construction
  line L126 (2123.7932, 2097.5746) -> (2095.9932, 2132.6055) construction
  line L127 (2077.1436, 2710.1377) -> (2112.7839, 2728.2973)
  line L128 (2112.7839, 2728.2973) -> (2121.8637, 2710.4772)
  line L129 (2121.8637, 2710.4772) -> (2086.2234, 2692.3176)
  line L130 (2086.2234, 2692.3176) -> (2077.1436, 2710.1377)
  line L131 (2077.1436, 2710.1377) -> (2121.8637, 2710.4772) construction
  line L132 (2112.7839, 2728.2973) -> (2086.2234, 2692.3176) construction
  line L133 (2018.0293, 2725.0702) -> (2047.2834, 2697.7902)
  line L134 (2047.2834, 2697.7902) -> (2060.9234, 2712.4173)
  line L135 (2060.9234, 2712.4173) -> (2031.6692, 2739.6972)
  line L136 (2031.6692, 2739.6972) -> (2018.0293, 2725.0702)
  line L137 (2018.0293, 2725.0702) -> (2060.9234, 2712.4173) construction
  line L138 (2047.2834, 2697.7902) -> (2031.6692, 2739.6972) construction
  line L139 (1612.0374, 2289.6972) -> (1641.2916, 2262.4173)
  line L140 (1641.2916, 2262.4173) -> (1627.6516, 2247.7902)
  line L141 (1627.6516, 2247.7902) -> (1598.3975, 2275.0702)
  line L142 (1598.3975, 2275.0702) -> (1612.0374, 2289.6972)
  line L143 (1612.0374, 2289.6972) -> (1627.6516, 2247.7902) construction
  line L144 (1641.2916, 2262.4173) -> (1598.3975, 2275.0702) construction
  line L145 (1613.7523, 2196.0764) -> (1631.8784, 2187.6241)
  line L146 (1631.8784, 2187.6241) -> (1648.7832, 2223.8764)
  line L147 (1648.7832, 2223.8764) -> (1630.657, 2232.3287)
  line L148 (1630.657, 2232.3287) -> (1613.7523, 2196.0764)
  line L149 (1613.7523, 2196.0764) -> (1648.7832, 2223.8764) construction
  line L150 (1631.8784, 2187.6241) -> (1630.657, 2232.3287) construction
  line L151 (2364.1848, 1327.5564) -> (2616.1835, 1867.9693) construction
  line L152 (2364.1848, 1327.5564) -> (2810.435, 953.108) construction
  line L153 (2571.8784, 1749.2949) -> (2588.7832, 1785.5472)
  line L154 (2588.7832, 1785.5472) -> (2570.657, 1793.9995)
  line L155 (2570.657, 1793.9995) -> (2553.7523, 1757.7472)
  line L156 (2553.7523, 1757.7472) -> (2571.8784, 1749.2949)
  line L157 (2571.8784, 1749.2949) -> (2570.657, 1793.9995) construction
  line L158 (2588.7832, 1785.5472) -> (2553.7523, 1757.7472) construction
  line L159 (2717.7978, 1017.7858) -> (2748.4396, 992.0743)
  line L160 (2748.4396, 992.0743) -> (2761.2953, 1007.3951)
  line L161 (2761.2953, 1007.3951) -> (2730.6535, 1033.1067)
  line L162 (2730.6535, 1033.1067) -> (2717.7978, 1017.7858)
  line L163 (2717.7978, 1017.7858) -> (2761.2953, 1007.3951) construction
  line L164 (2748.4396, 992.0743) -> (2730.6535, 1033.1067) construction
  line L165 (2532.7146, 1186.1431) -> (2239.6931, 1016.9671) construction
  line L166 (2276.5672, 1049.8034) -> (2311.2082, 1069.8034)
  line L167 (2311.2082, 1069.8034) -> (2321.2082, 1052.4829)
  line L168 (2321.2082, 1052.4829) -> (2286.5672, 1032.4829)
  line L169 (2286.5672, 1032.4829) -> (2276.5672, 1049.8034)
  line L170 (2276.5672, 1049.8034) -> (2321.2082, 1052.4829) construction
  line L171 (2311.2082, 1069.8034) -> (2286.5672, 1032.4829) construction
  line L172 (2207.2852, 1169.8034) -> (2241.9262, 1189.8034)
  line L173 (2241.9262, 1189.8034) -> (2251.9262, 1172.4829)
  line L174 (2251.9262, 1172.4829) -> (2217.2852, 1152.4829)
  line L175 (2217.2852, 1152.4829) -> (2207.2852, 1169.8034)
  line L176 (2207.2852, 1169.8034) -> (2251.9262, 1172.4829) construction
  line L177 (2241.9262, 1189.8034) -> (2217.2852, 1152.4829) construction
  line L178 (2127.0113, 1286.9462) -> (2145.1375, 1278.4939)
  line L179 (2145.1375, 1278.4939) -> (2128.2327, 1242.2416)
  line L180 (2128.2327, 1242.2416) -> (2110.1066, 1250.6939)
  line L181 (2110.1066, 1250.6939) -> (2127.0113, 1286.9462)
  line L182 (2127.0113, 1286.9462) -> (2128.2327, 1242.2416) construction
  line L183 (2145.1375, 1278.4939) -> (2110.1066, 1250.6939) construction
  line L184 (1477.0113, 1590.0462) -> (1495.1375, 1581.5939)
  line L185 (1495.1375, 1581.5939) -> (1478.2327, 1545.3415)
  line L186 (1478.2327, 1545.3415) -> (1460.1066, 1553.7939)
  line L187 (1460.1066, 1553.7939) -> (1477.0113, 1590.0462)
  line L188 (1477.0113, 1590.0462) -> (1478.2327, 1545.3415) construction
  line L189 (1495.1375, 1581.5939) -> (1460.1066, 1553.7939) construction
  line L190 (1065.9247, 1510.1391) -> (1095.1789, 1482.8592)
  line L191 (1095.1789, 1482.8592) -> (1081.5389, 1468.2321)
  line L192 (1081.5389, 1468.2321) -> (1052.2848, 1495.512)
  line L193 (1052.2848, 1495.512) -> (1065.9247, 1510.1391)
  line L194 (1065.9247, 1510.1391) -> (1081.5389, 1468.2321) construction
  line L195 (1095.1789, 1482.8592) -> (1052.2848, 1495.512) construction
  line L196 (694.4463, 1522.3354) -> (1002.9621, 1234.6398) construction
  line L197 (694.4463, 1522.3354) -> (363.0886, 1522.3354) construction
  line L198 (571.4463, 1693.5354) -> (355.5392, 1693.5354) construction
  line L199 (571.4463, 1693.5354) -> (656.7284, 1841.2483) construction
  line L200 (731.9463, 2243.3461) -> (543.0224, 2243.3461) construction
  line L201 (731.9463, 2243.3461) -> (906.1182, 2365.3025) construction
  line L202 (906.0454, 1338.6894) -> (935.2995, 1311.4095)
  line L203 (935.2995, 1311.4095) -> (921.6595, 1296.7824)
  line L204 (921.6595, 1296.7824) -> (892.4054, 1324.0624)
  line L205 (892.4054, 1324.0624) -> (906.0454, 1338.6894)
  line L206 (906.0454, 1338.6894) -> (921.6595, 1296.7824) construction
  line L207 (935.2995, 1311.4095) -> (892.4054, 1324.0624) construction
  line L208 (414.4463, 1532.3354) -> (374.4463, 1532.3354)
  line L209 (374.4463, 1532.3354) -> (374.4463, 1512.3354)
  line L210 (374.4463, 1512.3354) -> (414.4463, 1512.3354)
  line L211 (414.4463, 1512.3354) -> (414.4463, 1532.3354)
  line L212 (414.4463, 1532.3354) -> (374.4463, 1512.3354) construction
  line L213 (374.4463, 1532.3354) -> (414.4463, 1512.3354) construction
  line L214 (414.4463, 1703.5354) -> (374.4463, 1703.5354)
  line L215 (374.4463, 1703.5354) -> (374.4463, 1683.5354)
  line L216 (374.4463, 1683.5354) -> (414.4463, 1683.5354)
  line L217 (414.4463, 1683.5354) -> (414.4463, 1703.5354)
  line L218 (414.4463, 1703.5354) -> (374.4463, 1683.5354) construction
  line L219 (374.4463, 1703.5354) -> (414.4463, 1683.5354) construction
  line L220 (641.2861, 1834.5014) -> (661.2861, 1869.1424)
  line L221 (661.2861, 1869.1424) -> (678.6066, 1859.1424)
  line L222 (678.6066, 1859.1424) -> (658.6066, 1824.5014)
  line L223 (658.6066, 1824.5014) -> (641.2861, 1834.5014)
  line L224 (641.2861, 1834.5014) -> (678.6066, 1859.1424) construction
  line L225 (661.2861, 1869.1424) -> (658.6066, 1824.5014) construction
  line L226 (733.5066, 1781.2579) -> (753.5066, 1815.8989)
  line L227 (753.5066, 1815.8989) -> (736.1861, 1825.8989)
  line L228 (736.1861, 1825.8989) -> (716.1861, 1791.2579)
  line L229 (716.1861, 1791.2579) -> (733.5066, 1781.2579)
  line L230 (733.5066, 1781.2579) -> (736.1861, 1825.8989) construction
  line L231 (753.5066, 1815.8989) -> (716.1861, 1791.2579) construction
  line L232 (773.1861, 1889.9848) -> (790.5066, 1879.9848)
  line L233 (790.5066, 1879.9848) -> (770.5066, 1845.3438)
  line L234 (770.5066, 1845.3438) -> (753.1861, 1855.3438)
  line L235 (753.1861, 1855.3438) -> (773.1861, 1889.9848)
  line L236 (773.1861, 1889.9848) -> (770.5066, 1845.3438) construction
  line L237 (790.5066, 1879.9848) -> (753.1861, 1855.3438) construction
  line L238 (574.9463, 2253.3461) -> (534.9463, 2253.3461)
  line L239 (534.9463, 2253.3461) -> (534.9463, 2233.3461)
  line L240 (534.9463, 2233.3461) -> (574.9463, 2233.3461)
  line L241 (574.9463, 2233.3461) -> (574.9463, 2253.3461)
  line L242 (574.9463, 2253.3461) -> (534.9463, 2233.3461) construction
  line L243 (534.9463, 2253.3461) -> (574.9463, 2233.3461) construction
  line L244 (887.5835, 2364.5322) -> (854.8175, 2341.5891)
  line L245 (854.8175, 2341.5891) -> (866.289, 2325.2061)
  line L246 (866.289, 2325.2061) -> (899.0551, 2348.1491)
  line L247 (899.0551, 2348.1491) -> (887.5835, 2364.5322)
  line L248 (887.5835, 2364.5322) -> (866.289, 2325.2061) construction
  line L249 (854.8175, 2341.5891) -> (899.0551, 2348.1491) construction
  line L250 (940.4175, 2219.3397) -> (973.1835, 2242.2827)
  line L251 (973.1835, 2242.2827) -> (984.6551, 2225.8997)
  line L252 (984.6551, 2225.8997) -> (951.889, 2202.9566)
  line L253 (951.889, 2202.9566) -> (940.4175, 2219.3397)
  line L254 (940.4175, 2219.3397) -> (984.6551, 2225.8997) construction
  line L255 (973.1835, 2242.2827) -> (951.889, 2202.9566) construction
  line L256 (1032.2545, 2238.1521) -> (1061.5086, 2210.8721)
  line L257 (1061.5086, 2210.8721) -> (1047.8686, 2196.2451)
  line L258 (1047.8686, 2196.2451) -> (1018.6145, 2223.525)
  line L259 (1018.6145, 2223.525) -> (1032.2545, 2238.1521)
  line L260 (1032.2545, 2238.1521) -> (1047.8686, 2196.2451) construction
  line L261 (1061.5086, 2210.8721) -> (1018.6145, 2223.525) construction
  line L262 (1331.8545, 2559.4337) -> (1361.1086, 2532.1538)
  line L263 (1361.1086, 2532.1538) -> (1347.4686, 2517.5267)
  line L264 (1347.4686, 2517.5267) -> (1318.2145, 2544.8067)
  line L265 (1318.2145, 2544.8067) -> (1331.8545, 2559.4337)
  line L266 (1331.8545, 2559.4337) -> (1347.4686, 2517.5267) construction
  line L267 (1361.1086, 2532.1538) -> (1318.2145, 2544.8067) construction
  line L268 (1316.8819, 2582.9672) -> (1344.1618, 2612.2213)
  line L269 (1344.1618, 2612.2213) -> (1358.7889, 2598.5813)
  line L270 (1358.7889, 2598.5813) -> (1331.509, 2569.3272)
  line L271 (1331.509, 2569.3272) -> (1316.8819, 2582.9672)
  line L272 (1316.8819, 2582.9672) -> (1358.7889, 2598.5813) construction
  line L273 (1344.1618, 2612.2213) -> (1331.509, 2569.3272) construction
  line L274 (1215.7618, 2731.9563) -> (1188.4819, 2702.7021)
  line L275 (1188.4819, 2702.7021) -> (1203.109, 2689.0621)
  line L276 (1203.109, 2689.0621) -> (1230.3889, 2718.3163)
  line L277 (1230.3889, 2718.3163) -> (1215.7618, 2731.9563)
  line L278 (1215.7618, 2731.9563) -> (1203.109, 2689.0621) construction
  line L279 (1188.4819, 2702.7021) -> (1230.3889, 2718.3163) construction
  line L280 (1174.2015, 2740.4491) -> (1194.2015, 2740.4491)
  line L281 (1194.2015, 2740.4491) -> (1194.2015, 2700.4491)
  line L282 (1194.2015, 2700.4491) -> (1174.2015, 2700.4491)
  line L283 (1174.2015, 2700.4491) -> (1174.2015, 2740.4491)
  line L284 (1174.2015, 2740.4491) -> (1194.2015, 2700.4491) construction
  line L285 (1194.2015, 2740.4491) -> (1174.2015, 2700.4491) construction
  line L286 (845.5626, 2740.4491) -> (865.5626, 2740.4491)
  line L287 (865.5626, 2740.4491) -> (865.5626, 2700.4491)
  line L288 (865.5626, 2700.4491) -> (845.5626, 2700.4491)
  line L289 (845.5626, 2700.4491) -> (845.5626, 2740.4491)
  line L290 (845.5626, 2740.4491) -> (865.5626, 2700.4491) construction
  line L291 (865.5626, 2740.4491) -> (845.5626, 2700.4491) construction
  line L292 (303.5626, 2158.4491) -> (263.5626, 2158.4491)
  line L293 (263.5626, 2158.4491) -> (263.5626, 2138.4491)
  line L294 (263.5626, 2138.4491) -> (303.5626, 2138.4491)
  line L295 (303.5626, 2138.4491) -> (303.5626, 2158.4491)
  line L296 (303.5626, 2158.4491) -> (263.5626, 2138.4491) construction
  line L297 (263.5626, 2158.4491) -> (303.5626, 2138.4491) construction
  line L298 (213.5626, 1345.9491) -> (213.5626, 845.9491) construction
  line L299 (213.5626, 845.9491) -> (100.8718, 845.9491) construction
  line L300 (213.5626, 1345.9491) -> (213.5626, 1845.9491) construction
  line L301 (213.5626, 1845.9491) -> (119.6712, 1845.9491) construction
  line L302 (123.5626, 1835.9491) -> (163.5626, 1835.9491)
  line L303 (163.5626, 1835.9491) -> (163.5626, 1855.9491)
  line L304 (163.5626, 1855.9491) -> (123.5626, 1855.9491)
  line L305 (123.5626, 1855.9491) -> (123.5626, 1835.9491)
  line L306 (123.5626, 1835.9491) -> (163.5626, 1855.9491) construction
  line L307 (163.5626, 1835.9491) -> (123.5626, 1855.9491) construction
  line L308 (163.5626, 855.9491) -> (123.5626, 855.9491)
  line L309 (123.5626, 855.9491) -> (123.5626, 835.9491)
  line L310 (123.5626, 835.9491) -> (163.5626, 835.9491)
  line L311 (163.5626, 835.9491) -> (163.5626, 855.9491)
  line L312 (163.5626, 855.9491) -> (123.5626, 835.9491) construction
  line L313 (123.5626, 855.9491) -> (163.5626, 835.9491) construction
  point P0 (0, 0)
  point P1 (283.5626, 543.4491)
  point P2 (440.0099, 412.1742)
  point P3 (708.1888, 352.7204)
  point P4 (958.2337, 330.8443)
  point P5 (1208.2337, 447.4212)
  point P6 (1231.3057, 510.811)
  point P7 (1459.6046, 869.1685)
  point P8 (1523.8046, 869.1685)
  point P9 (1558.5733, 918.8233)
  point P10 (1722.8515, 1203.3615)
  point P11 (1752.8644, 1246.2244)
  point P12 (1772.1938, 1390.8841)
  point P13 (2109.8932, 2115.0901)
  point P14 (2099.5036, 2710.3074)
  point P15 (2039.4763, 2718.7437)
  point P16 (1619.8445, 2268.7437)
  point P17 (1631.2677, 2209.9764)
  point P18 (2571.2677, 1771.6472)
  point P19 (2739.5466, 1012.5905)
  point P20 (2298.8877, 1051.1431)
  point P21 (2229.6057, 1171.1431)
  point P22 (2127.622, 1264.5939)
  point P23 (1477.622, 1567.6939)
  point P24 (1073.7318, 1489.1856)
  point P25 (913.8525, 1317.7359)
  point P26 (394.4463, 1522.3354)
  point P27 (394.4463, 1693.5354)
  point P28 (659.9463, 1846.8219)
  point P29 (734.8463, 1803.5784)
  point P30 (771.8463, 1867.6643)
  point P31 (554.9463, 2243.3461)
  point P32 (876.9363, 2344.8691)
  point P33 (962.5363, 2222.6197)
  point P34 (1040.0615, 2217.1986)
  point P35 (1339.6615, 2538.4802)
  point P36 (1337.8354, 2590.7743)
  point P37 (1209.4354, 2710.5092)
  point P38 (1184.2015, 2720.4491)
  point P39 (855.5626, 2720.4491)
  point P40 (283.5626, 2148.4491)
  point P41 (143.5626, 1845.9491)
  point P42 (143.5626, 845.9491)
  dimension "d159" = 40
  dimension "d160" = 20
  dimension "d161" = 50
  dimension "d162" = 20
  dimension "d163" = 40
  dimension "d164" = 50
  dimension "d165" = 20
  dimension "d166" = 40
  dimension "d167" = 50
  dimension "d168" = 20
  dimension "d169" = 40
  dimension "d170" = 50
  dimension "d171" = 20
  dimension "d172" = 40
  dimension "d173" = 50
  dimension "d174" = 40
  dimension "d175" = 20
  dimension "d176" = 50
  dimension "d177" = 20
  dimension "d178" = 40
  dimension "d179" = 50
  dimension "d180" = 20
  dimension "d181" = 40
  dimension "d182" = 50
  dimension "d183" = 40
  dimension "d184" = 20
  dimension "d185" = 50
  dimension "d186" = 20
  dimension "d187" = 40
  dimension "d188" = 50
  dimension "d189" = 40
  dimension "d190" = 20
  dimension "d191" = 50
  dimension "d192" = 40
  dimension "d193" = 20
  dimension "d194" = 50
  dimension "d195" = 40
  dimension "d196" = 20
  dimension "d197" = 50
  dimension "d198" = 40
  dimension "d199" = 20